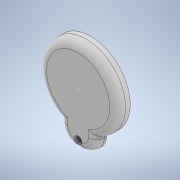
# Autodesk Inventor part: fixedpart
Saved by Autodesk Inventor 2021 (Build 250183000, 183)
## iProperties
Created: 2021-03-16
Part Number: fixedpart
Material: Generic
Document SubType Name: Modeling
Designer: Olivi
Density: 1 g/cm^3
Appearance: Default
Author: Olivi
Autodesk Inventor part; units mm, degrees
ref_plane "YZ Plane" through (0, 0, 0) normal (1, 0, 0) x (0, 1, 0)
ref_plane "XZ Plane" through (0, 0, 0) normal (0, 1, 0) x (-1, 0, 0)
ref_plane "XY Plane" through (0, 0, 0) normal (0, 0, 1) x (1, 0, 0)
sketch "Sketch1" plane through (0, 0, 0) normal (0, 0, 1) x (1, 0, 0)
  circle A0 centre (0, 0) radius 3.95
  dimension "d0" = 7.9
  constraints: 1 centre point, 1 coincident
  measures "d0" diameter of A0
extrude "Extrusion1" add sketch "Sketch1" along normal blind 7
sketch "Sketch2" plane through (0, 0, 7) normal (0, 0, 1) x (1, 0, 0)
  circle A0 centre (0, 0) radius 25
  dimension "d3" = 50
  constraints: 1 centre point, 1 coincident
  measures "d3" diameter of A0
extrude "Extrusion2" add sketch "Sketch2" along normal blind 8
sketch "Sketch3" plane through (0, 0, 15) normal (0, 0, 1) x (1, 0, 0)
  point P0 (0, 0)
sketch "Sketch5" plane through (0, 0, 15) normal (0, 0, 1) x (1, 0, 0)
  line L0 (-11.5, -16.5) -> (11.5, -16.5)
  line L1 (11.5, -16.5) -> (11.5, -33.5)
  line L2 (11.5, -33.5) -> (-11.5, -33.5)
  line L3 (-11.5, -33.5) -> (-11.5, -16.5)
  circle A0 centre (0, 0) radius 25
  line L4 (-11.5, -16.5) -> (11.5, -33.5) construction
  line L5 (11.5, -16.5) -> (-11.5, -33.5) construction
  arc A1 (-11.5, -22.198) -> (11.5, -22.198) centre (0, 0) ccw
  point P0 (0, -25)
  dimension "d8" = 23
  dimension "d12" = 17
  dimension "d13" = 0
  dimension "d14" = 50
  constraints: 12 end point, 6 point on circle, 2 centre point, 2 midpoint, 2 parallel, 2 point on line, 1 horizontal, 1 perpendicular
  measures "d8" distance of L1.end L2.end
  measures "d12" distance of L2.end L0.start
  measures "d13" distance of point (0, 0) A0.centre
  measures "d14" diameter of A0
extrude "Extrusion4" add sketch "Sketch5" against normal blind 6.5 contours A0 L1 L2 L3
fillet "Fillet1" radius 10 2 edges at (-11.5, -33.5, 11.75) (11.5, -33.5, 11.75)
sketch "Sketch6" plane through (0, 0, 15) normal (0, 0, 1) x (1, 0, 0)
  circle A0 centre (0, -28) radius 2.25
  line L0 (-1.5, -33.5) -> (1.5, -33.5) projected
  point P0 (0, 0)
  dimension "d15" = 4.5
  dimension "d16" = 5.5
  constraints: 1 centre point
  measures "d15" diameter of A0
  measures "d16" distance from line of L0 A0.centre
extrude "Extrusion5" cut sketch "Sketch6" against normal through all
fillet "Fillet2" radius 5 7 edges at (-12.9904, 21.36, 15) (21.36, -12.9904, 15) (-11.5, -22.849, 15) (0, -33.5, 15) (8.5711, -30.5711, 15) (11.5, -22.849, 15) (-8.5711, -30.5711, 15)
body "Solid1"
